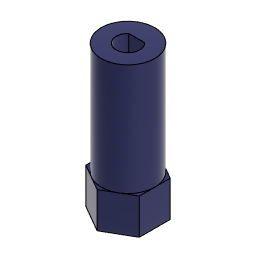
Coupler v8 (Autodesk Fusion 360 design; units mm, degrees)
Autodesk Fusion 360 part; units mm, degrees
form "Form1" [no effect]
sketch "sketch 223" plane through (0, 0, 0) normal (0, 0, 1) x (1, 0, 0)
  line L0 (12, 6.9282) -> (0, 13.8564)
  line L1 (0, 13.8564) -> (-12, 6.9282)
  line L2 (-12, 6.9282) -> (-12, -6.9282)
  line L3 (-12, -6.9282) -> (0, -13.8564)
  line L4 (0, -13.8564) -> (12, -6.9282)
  line L5 (12, -6.9282) -> (12, 6.9282)
extrude "Extrude1" add sketch "sketch 223" along normal blind 8
sketch "Sketch1" plane through (0, 0, 8) normal (0, 0, 1) x (-1, 0, 0)
  line L0 (-12, 6.9282) -> (-12, -6.9282)
  line L1 (-12, -6.9282) -> (0, -13.8564)
  line L2 (0, -13.8564) -> (12, -6.9282)
  line L3 (12, -6.9282) -> (12, 6.9282)
  line L4 (12, 6.9282) -> (0, 13.8564)
  line L5 (0, 13.8564) -> (-12, 6.9282)
  circle A0 centre (0, 0) radius 12
  constraint coincident A0.centre origin
  constraint tangent L3 A0
extrude "Extrude2" add sketch "Sketch1" along normal blind 25 contours A0
sketch "Sketch2" plane through (0, 0, 33) normal (0, 0, 1) x (-1, 0, 0)
  circle A0 centre (0, 0) radius 12
  circle A1 centre (0, 0) radius 2.65
  line L0 (0, 0) -> (0, 2.65)
  line L1 (0, 2.65) -> (0, -1.95)
  line L2 (0, -1.95) -> (-1.7944, -1.95)
  line L3 (0, -1.95) -> (1.7944, -1.95)
  circle A2 centre (0, 0) radius 6
  dimension "d5" = 5.3
  dimension "d6" = 4.6
  dimension "d20" = 12
  constraint coincident A0.centre A1.centre
  constraint coincident A1 L0.end
  constraint vertical L0
  constraint parallel L0 L1
  constraint coincident A1 L2.end
  constraint perpendicular L0 L2
  constraint coincident A1 L3.end
  constraint perpendicular L1 L3
  measures "d5" diameter of A1
  measures "d6" distance of L0.end L1.end
  measures "d20" diameter of A2
extrude "Extrude3" cut sketch "Sketch2" against normal blind 25 contours A1 L0 L1 L3 | A1 L0 L1 L2
sketch "Sketch3" plane through (0, 0, 0) normal (0, 0, -1) x (1, 0, 0)
  line L0 (12, -6.9282) -> (12, 6.9282)
  line L1 (12, 6.9282) -> (0, 13.8564)
  line L2 (0, 13.8564) -> (-12, 6.9282)
  line L3 (-12, 6.9282) -> (-12, -6.9282)
  line L4 (-12, -6.9282) -> (0, -13.8564)
  line L5 (0, -13.8564) -> (12, -6.9282)
  circle A0 centre (0, 0) radius 2.5
  dimension "d9" = 5
  constraint coincident A0.centre origin
  measures "d9" diameter of A0
extrude "Extrude4" cut sketch "Sketch3" against normal blind 8 contours A0
sketch "Sketch5" plane through (0, 1.95, 0) normal (0, -1, 0) x (1, 0, 0)
  line L0 (1.7944, 33) -> (-1.7944, 33)
  line L1 (-1.7944, 33) -> (-1.7944, 8)
  line L2 (-1.5644, 8) -> (1.5644, 8)
  line L3 (1.7944, 8) -> (1.7944, 33)
  line L4 (0, 19) -> (0, 8)
  line L5 (0, 33) -> (1.5644, 33)
  line L6 (1.5644, 33) -> (1.5644, 8)
  line L7 (1.5644, 8) -> (0, 8)
  line L8 (0, 19) -> (1.5644, 19)
  line L9 (0, 13.5) -> (1.7944, 13.5)
  circle A0 centre (0, 13.5) radius 2
  circle A1 centre (0, 24.5) radius 2
  line L10 (-1.7944, 8) -> (-1.5644, 8)
  line L11 (1.5644, 8) -> (1.7944, 8)
  dimension "d12" = 4
  constraint midpoint L0 L5.start
  constraint midpoint L2 L4.end
  constraint perpendicular L3 L5
  constraint coincident L2.end L6.end
  constraint perpendicular L2 L6
  constraint coincident L6 L8.end
  constraint perpendicular L6 L8
  constraint midpoint L4 L9.start
  constraint coincident L3 L9.end
  constraint perpendicular L3 L9
  constraint coincident L9.start A0.centre
  constraint symmetric L8 A0 A1
  measures "d12" diameter of A0
extrude "Extrude5" cut sketch "Sketch5" against normal blind 11 contours L3 A1 | L3 L6 A1 | L1 L6 A1 | L1 A1 | L3 A0 | L3 L6 L9 A0 | L3 L6 L9 A0 | L4 L6 L9 A0 | L1 L4 A0 | L1 A0 | L4 L6 L9 A0
extrude "Extrude6" cut sketch "Sketch5" along normal blind 1.5 contours L3 A1 | L3 L6 A1 | L1 L6 A1 | L1 A1 | L3 A0 | L3 L6 L9 A0 | L3 L6 L9 A0 | L4 L6 L9 A0 | L1 L4 A0 | L1 A0 | L4 L6 L9 A0
sketch "Sketch6" plane through (0, 0, 0) normal (0, 0, 1) x (1, 0, 0)
  line L0 (6, 3.4641) -> (0, 6.9282)
  line L1 (0, 6.9282) -> (-6, 3.4641)
  line L2 (-6, 3.4641) -> (-6, -3.4641)
  line L3 (-6, -3.4641) -> (0, -6.9282)
  line L4 (0, -6.9282) -> (6, -3.4641)
  line L5 (6, -3.4641) -> (6, 3.4641)
  line L6 (-15, -15) -> (15, -15)
  line L7 (15, -15) -> (15, 15)
  line L8 (15, 15) -> (-15, 15)
  line L9 (-15, 15) -> (-15, -15)
  dimension "d17" = 6
  constraint horizontal L6
  constraint vertical L7
  constraint horizontal L8
  constraint vertical L9
  measures "d17" distance of origin L5
extrude "Extrude7" cut sketch "Sketch6" along normal blind 8
extrude "Extrude8" cut sketch "Sketch2" against normal blind 25 contours A0
